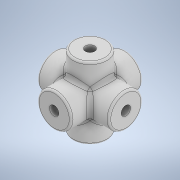
# Autodesk Inventor part: rubix
Saved by Autodesk Inventor 2020 (Build 240168000, 168)
## iProperties
Created: 2019-09-30
Part Number: rubix
Material: Generic
Document SubType Name: Modeling
Designer: eduso287260
Density: 1 g/cm^3
Appearance: Default
Author: eduso287260
Autodesk Inventor part; units mm, degrees
ref_plane "YZ Plane" through (0, 0, 0) normal (1, 0, 0) x (0, 1, 0)
ref_plane "XZ Plane" through (0, 0, 0) normal (0, 1, 0) x (-1, 0, 0)
ref_plane "XY Plane" through (0, 0, 0) normal (0, 0, 1) x (1, 0, 0)
sketch "Sketch2" plane through (0, 0, 0) normal (1, 0, 0) x (0, 1, 0)
  circle A0 centre (0, 0) radius 4.5
  dimension "d1" = 9
  constraints: 1 centre point
  measures "d1" diameter of A0
extrude "Extrusion1" add sketch "Sketch2" along normal mid plane 19
sketch "Sketch4" plane through (0, 0, 0) normal (0, 1, 0) x (-1, 0, 0)
  circle A0 centre (0, 0) radius 4.5
  dimension "d5" = 9
  constraints: 1 centre point, 1 coincident
  measures "d5" diameter of A0
extrude "Extrusion2" add sketch "Sketch4" along normal mid plane 19
sketch "Sketch5" plane through (0, 0, 0) normal (0, 0, 1) x (1, 0, 0)
  circle A0 centre (0, 0) radius 4.5
  line L0 (0, 0) -> (-4.5, -4.5) projected
  dimension "d10" = 9
  constraints: 1 centre point, 1 coincident
  measures "d10" diameter of A0
extrude "Extrusion3" add sketch "Sketch5" along normal mid plane 19
sketch "Sketch6" plane through (0, 9.5, 0) normal (0, 1, 0) x (1, 0, 0)
  point P0 (0, 0)
  point P1 (0, 0)
  constraints: 1 coincident
hole "Hole1" at (0, 9.5, 0) direction (0, -1, 0) diameter 2.5 depth 20 tip angle 118
sketch "Sketch7" plane through (0, 0, 9.5) normal (0, 0, 1) x (1, 0, 0)
  point P0 (0, 0)
  point P1 (0, 0)
  constraints: 1 coincident
hole "Hole2" at (0, 0, 9.5) direction (0, 0, -1) diameter 2.5 depth 20 tip angle 118
sketch "Sketch8" plane through (9.5, 0, 0) normal (1, 0, 0) x (0, 0, -1)
  point P0 (0, 0)
  point P1 (0, 0)
  constraints: 1 coincident
hole "Hole3" at (9.5, 0, 0) direction (-1, 0, 0) diameter 2.5 depth 20 tip angle 118
fillet "Fillet4" radius 0.5 6 edges at (4.5, 9.5, 0) (-9.5, -4.5, 0) (-4.5, 0, -9.5) (9.5, -4.5, 0) (-4.5, 0, 9.5) (4.5, -9.5, 0)
fillet "Fillet5" radius 1 17 edges at (0, 4.5, 4.5) (-4.5, 0, 4.5) (-4.1575, 4.1575, -1.7221) (-4.1575, 4.1575, 1.7221) (0, 4.5, -4.5) (-4.5, 0, -4.5) (-4.1575, -4.1575, -1.7221) (-4.1575, -4.1575, 1.7221) (0, -4.5, -4.5) (4.1575, 1.7221, -4.1575) (4.1575, -1.7221, -4.1575) (4.5, -4.5, 0) (4.1575, 1.7221, 4.1575) (4.1575, -1.7221, 4.1575) (0, -4.5, 4.5) (4.1575, 4.1575, -1.7221) (4.1575, 4.1575, 1.7221)
body "Solid1"
